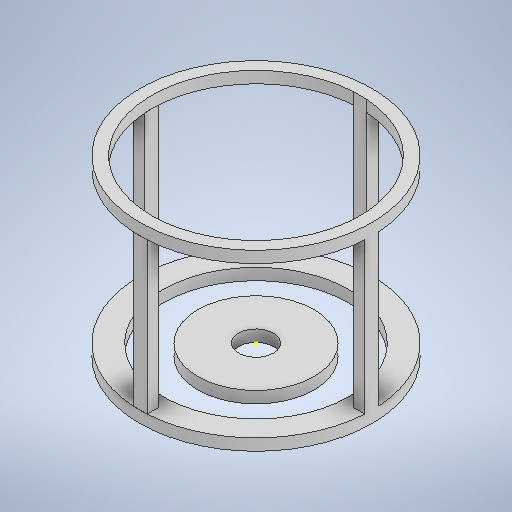
# Autodesk Inventor part: Walec2
Saved by Autodesk Inventor 2025 (Build 290162000, 162)
## iProperties
Created: 2024-12-31
Part Number: Walec2
Material: Ogólny
Document SubType Name: Modeling
Designer: Laptop
Density: 1 g/cm^3
Appearance: Domyślna
Author: Laptop
Autodesk Inventor part; units mm, degrees
ref_plane "YZ Plane" through (0, 0, 0) normal (1, 0, 0) x (0, 1, 0)
ref_plane "XZ Plane" through (0, 0, 0) normal (0, 1, 0) x (-1, 0, 0)
ref_plane "XY Plane" through (0, 0, 0) normal (0, 0, 1) x (1, 0, 0)
sketch "Szkic1" plane through (0, 0, 0) normal (0, 1, 0) x (-1, 0, 0)
  circle A0 centre (0, 0) radius 50
  dimension "d0" = 100
  constraints: 1 centre point, 1 coincident
  measures "d0" diameter of A0
extrude "Wyciągnięcie proste1" add sketch "Szkic1" along normal blind 80
sketch "Szkic2" plane through (0, 80, 0) normal (0, 1, 0) x (1, 0, 0)
  circle A0 centre (0, 0) radius 45
  dimension "d3" = 90
  constraints: 1 centre point, 1 coincident
  measures "d3" diameter of A0
extrude "Wyciągnięcie proste2" cut sketch "Szkic2" against normal blind 75
sketch "Szkic3" plane through (0, 5, 0) normal (0, 1, 0) x (1, 0, 0)
  point P0 (0, 0)
sketch "Szkic4" plane through (0, 5, 0) normal (0, 1, 0) x (1, 0, 0)
  circle A0 centre (0, 0) radius 7.5
  dimension "d6" = 15
  constraints: 1 centre point, 1 coincident
  measures "d6" diameter of A0
extrude "Wyciągnięcie proste3" cut sketch "Szkic4" against normal blind 75
sketch "Szkic9" plane through (0, 80, 0) normal (0, 1, 0) x (1, 0, 0)
  circle A0 centre (0, 0) radius 50 projected
  line L0 (-49.9099, 3) -> (-44.8999, 3)
  circle A1 centre (0, 0) radius 45 projected
  line L1 (-49.9099, -3) -> (-44.8999, -3)
  line L2 (44.9005, 2.9912) -> (49.9104, 2.9912)
  line L3 (44.6345, -3) -> (49.9099, -3)
  arc A2 (-49.9099, -3) -> (49.9099, -3) centre (0, 0) ccw
  arc A3 (-40.5012, -19.6125) -> (44.6345, -3) centre (-0.1275, -0.0618) ccw
  arc A4 (49.9104, 2.9912) -> (-49.9099, 3) centre (0, 0) ccw
  arc A5 (44.9005, 2.9912) -> (-44.8999, 3) centre (-0.0001, -0.7186) ccw
  point P0 (44.9005, 2.9912)
  point P1 (44.8999, -3)
  constraints: 14 point on circle, 8 end point, 4 centre point, 4 horizontal, 2 concentric, 1 tangent
extrude "Wyciągnięcie proste4" cut sketch "Szkic9" against normal blind 75 contours L2 A1 L0 A0 | A0 L1 A1 L3
sketch "Szkic10" plane through (0, 80, 0) normal (0, 1, 0) x (1, 0, 0)
  circle A0 centre (0, 0) radius 50
  arc A1 (44.8999, -3) -> (44.9005, 2.9912) centre (0, 0) ccw projected
  circle A2 centre (0, 0) radius 45
  point P0 (44.9005, 2.9912)
  constraints: 2 coincident, 1 centre point, 3 other
extrude "Wyciągnięcie proste5" cut sketch "Szkic10" against normal blind 10
sketch "Szkic11" plane through (0, 70, 0) normal (0, 1, 0) x (1, 0, 0)
  circle A0 centre (0, 0) radius 7.5 projected
  circle A1 centre (0, 0) radius 50
  circle A2 centre (0, 0) radius 44.8999
  constraints: 2 centre point, 2 coincident
extrude "Wyciągnięcie proste6" add sketch "Szkic11" along normal blind 5 contours A1
sketch "Szkic12" plane through (0, 5, 0) normal (0, 1, 0) x (1, 0, 0)
  circle A0 centre (0, 0) radius 44.8999 projected
  circle A1 centre (0, 0) radius 50 projected
  line L0 (-3, -44.7996) -> (3, -44.7996)
  line L1 (3, -44.7996) -> (3, -49.9099)
  line L2 (3, -49.9099) -> (-3, -49.9099)
  line L3 (-3, -49.9099) -> (-3, -44.7996)
  dimension "d20" = 6
  constraints: 8 end point, 2 parallel, 1 horizontal, 1 perpendicular, 4 other
  measures "d20" distance of L1.end L2.end
extrude "Wyciągnięcie proste7" add sketch "Szkic12" along normal blind 70 contours A0 L1 L2 L3
sketch "Szkic13" plane through (0, 5, 0) normal (0, 1, 0) x (1, 0, 0)
  arc A0 (3, -44.7996) -> (-3, -44.7996) centre (0, 0) ccw projected
  arc A1 (49.9104, 2.9912) -> (-49.9099, 3) centre (0, 0) ccw projected
  line L0 (-3, 44.7996) -> (3, 44.7996)
  line L1 (3, 44.7996) -> (3, 49.9099)
  line L2 (3, 49.9099) -> (-3, 49.9099)
  line L3 (-3, 49.9099) -> (-3, 44.7996)
  dimension "d23" = 6
  constraints: 8 end point, 2 parallel, 2 point on circle, 1 horizontal, 1 perpendicular
  measures "d23" distance of L2.end L1.end
extrude "Wyciągnięcie proste8" add sketch "Szkic13" along normal blind 70 contours L0 A0 | A0 L3 L2 L1
sketch "Szkic14" plane through (0, 5, 0) normal (0, 1, 0) x (1, 0, 0)
  circle A0 centre (0, 0) radius 7.5 projected
  circle A1 centre (0, 0) radius 25
  circle A2 centre (0, 0) radius 40
  dimension "d26" = 50
  dimension "d27" = 80
  constraints: 2 centre point, 2 coincident
  measures "d26" diameter of A1
  measures "d27" diameter of A2
extrude "Wyciągnięcie proste9" cut sketch "Szkic14" against normal blind 70 contours A2
